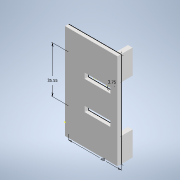
# Autodesk Inventor part: Encoderadapter
Saved by Autodesk Inventor 2022 (Build 260153070, 153G)
## iProperties
Created: 2021-11-29
Part Number: Encoderadapter
Material: Generic
Document SubType Name: Modeling
Designer: a laptop
Density: 1 g/cm^3
Appearance: Default
Mass: 8.1788 g
Surface Area: 69.1009 cm^2
Volume: 8.1788 cm^3
Author: a laptop
Autodesk Inventor part; units mm, degrees
ref_plane "YZ Plane" through (0, 0, 0) normal (1, 0, 0) x (0, 1, 0)
ref_plane "XZ Plane" through (0, 0, 0) normal (0, 1, 0) x (-1, 0, 0)
sketch "Sketch1" plane through (0, 0, 0) normal (0, 0, 1) x (1, 0, 0)
  line L0 (0, 44.8) -> (0, 9.25)
  line L1 (0, 44.8) -> (40, 44.8)
  line L2 (0, 9.25) -> (40, 9.25)
  line L3 (40, 9.25) -> (40, 44.8)
  line L4 (14.9707, 35.95) -> (34.6293, 35.95)
  line L5 (34.6293, 35.95) -> (34.6293, 40.05)
  line L6 (34.6293, 40.05) -> (14.9707, 40.05)
  line L7 (14.9707, 40.05) -> (14.9707, 35.95)
  line L8 (30.8793, 39.05) -> (28.5722, 39.05) construction
  line L9 (30.8793, 39.05) -> (30.8793, 36.95) construction
  line L10 (30.8793, 36.95) -> (28.5722, 36.95) construction
  line L11 (28.5722, 39.05) -> (28.5722, 36.95) construction
  line L12 (30.8793, 39.05) -> (30.8793, 40.05) construction
  line L13 (30.8793, 36.95) -> (30.8793, 35.95) construction
  line L14 (21.0278, 39.05) -> (18.7207, 39.05) construction
  line L15 (21.0278, 39.05) -> (21.0278, 36.95) construction
  line L16 (21.0278, 36.95) -> (18.7207, 36.95) construction
  line L17 (18.7207, 39.05) -> (18.7207, 36.95) construction
  line L18 (18.7207, 39.05) -> (14.9707, 39.05) construction
  line L19 (30.8793, 39.05) -> (34.6293, 39.05) construction
  line L20 (0, -9.25) -> (0, 9.25) projected
  line L21 (40, 27.025) -> (0, 27.025) construction
  line L22 (14.9707, 18.1) -> (34.6293, 18.1)
  line L23 (34.6293, 18.1) -> (34.6293, 14)
  line L24 (34.6293, 14) -> (14.9707, 14)
  line L25 (14.9707, 14) -> (14.9707, 18.1)
  line L26 (40, 9.25) -> (40, -9.25)
  line L27 (40, -9.25) -> (0, -9.25)
  line L28 (32.375, -9.25) -> (32.375, 9.25) projected
  line L29 (36.5, 9.25) -> (36.5, -9.3) projected
  line L30 (0, 44.8) -> (40, 44.8)
  line L31 (0, 63.3) -> (0, 44.8)
  line L32 (40, 44.8) -> (40, 63.3)
  line L33 (40, 63.3) -> (0, 63.3)
  line L34 (32.375, 63.3) -> (32.375, 44.8)
  line L35 (36.5, 44.8) -> (36.5, 63.35)
  point P0 (36.5, -9.25)
  point P1 (36.5, 63.3)
  dimension "d1" = 35.55
  dimension "d2" = 1
  dimension "d3" = 3.75
  dimension "d4" = 40
  constraints: 50 end point, 11 symmetric about line, 6 point on line, 5 perpendicular, 3 horizontal, 3 parallel, 2 collinear, 2 midpoint, 2 vertical, 1 coincident, 1 horizontal alignment, 1 other
  measures "d1" distance of L0.start L0.end
  measures "d2" distance of L9.end L13.end
  measures "d3" distance of L8.start L19.end
  measures "d4" distance of L26.end L20.start
extrude "Extrusion1" add sketch "Sketch1" along normal blind 2.75
ref_plane "Work Plane1" through (36.5, 52.55, -8.75) normal (0, 0, 1) x (1, 0, 0)
extrude "Extrusion2" add sketch "Sketch1" against normal up to surface (8.75 mm away) contours L35 L33 L32 L1 | L2 L26 L27 L29
ref_plane "Work Plane2" through (27.7797, 32.4377, -8.357) normal (-0.3827, 0, -0.9239) x (-0.4619, -0.866, 0.1913)
sketch "Sketch3" plane through (27.7797, 32.4377, -8.357) normal (-0.3827, 0, -0.9239) x (-0.4619, -0.866, 0.1913)
  circle A0 centre (5.5343, -1.2396) radius 6.25 construction
  ellipse E0 centre (5.5343, -1.2396) end of major axis (-0.7444, 2.3854) minor radius 7.25
  line L0 (10.947, -4.3646) -> (11.813, -4.8646) construction
  line L1 (2.4093, -6.6522) -> (1.9093, -7.5183) construction
  line L2 (0.6415, -9.7142) -> (19.1191, 22.2899) construction
  point P0 (42.5234, 8.7774)
  dimension "d9" = 1
  constraints: 4 end point, 2 line through centre, 2 perpendicular, 2 point on circle, 1 coincident, 6 other
  measures "d9" distance of L0.start L0.end
extrude "Extrusion3" cut sketch "Sketch3" against normal blind 17.75
body "Solid1"
